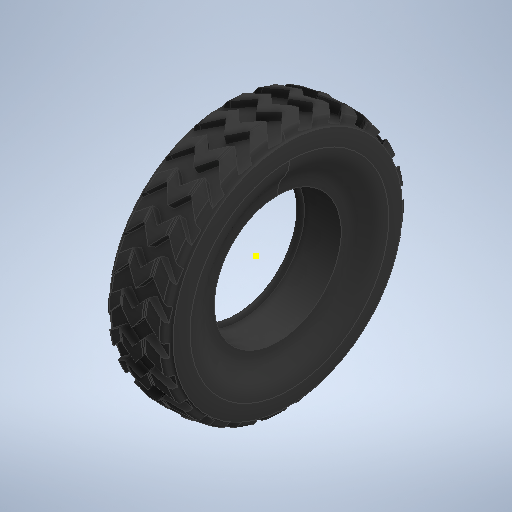
# Autodesk Inventor part: eg 243 tyre
Saved by Autodesk Inventor 2025 (Build 290162000, 162)
## iProperties
Created: 2024-11-03
Part Number: eg 243 tyre
Material: Generic
Document SubType Name: Modeling
Designer: Student
Density: 1 g/cm^3
Appearance: Default
Author: Student
Autodesk Inventor part; units mm, degrees
ref_plane "YZ Plane" through (0, 0, 0) normal (1, 0, 0) x (0, 1, 0)
ref_plane "XZ Plane" through (0, 0, 0) normal (0, 1, 0) x (-1, 0, 0)
sketch "Sketch1" plane through (0, 0, 0) normal (0, 0, 1) x (1, 0, 0)
  line L0 (65, 190) -> (-45, 190)
  arc A0 (75, 397) -> (-75, 397) centre (0, 49.4375) ccw
  arc A1 (-75, 397) -> (-100, 297.5) centre (110.505, 297.5) ccw
  spline S0 degree 4 poles (-100, 297.5) (-100, 283.0211) (-97.3443, 254.0633) (-65, 233.4367) (-65, 204.4789) (-65, 190) knots 0 0 0 0 0 0.5 1 1 1 1 1
  arc A2 (100, 297.5) -> (75, 397) centre (-110.505, 297.5) ccw
  arc A3 (-65, 190) -> (-45, 190) centre (-55, 190) ccw
  line L1 (-45, 190) -> (65, 190)
  line L2 (-75, 0) -> (75, 0)
  line L3 (65, 190) -> (65, 219.4167)
  spline S1 degree 4 poles (100, 297.5) (100, 283.0211) (97.3443, 254.0633) (65, 233.4367) (65, 204.4789) (65, 190) knots 0 0 0 0 0 0.5 1 1 1 1 1
  point P0 (0, 0)
  dimension "d11" = 20
  constraints: 8 end point, 8 point on circle, 4 centre point, 2 vertical, 1 collinear, 1 horizontal, 7 other
  measures "d11" distance of A3.start L0.end
revolve "Revolution1" add sketch "Sketch1" angle 360 about axis through (-75, 0, 0) along (1, 0, 0)
sketch "Sketch2" plane through (0, 0, 0) normal (0, 0, 1) x (1, 0, 0)
  line L0 (0, 0) -> (0, 447.3239)
  line L1 (0, 0) -> (252.2456, 0)
  line L2 (-125.0211, 343.2156) -> (-94.976, 343.2156)
  arc A0 (-75, 397) -> (-100, 297.5) centre (110.505, 297.5) ccw projected
  line L3 (-75, -397) -> (-75, 397) projected
  line L4 (-75, 364.2118) -> (-38.26, 370.6901)
  arc A1 (-38.26, 370.6901) -> (-34.9982, 371.8769) centre (-39.9965, 380.5381) ccw
  arc A2 (-30, 373.2156) -> (-34.9982, 371.8769) centre (-30, 363.2156) ccw
  line L5 (-30, 373.2156) -> (0, 373.2156)
  spline S0 degree 4 poles (-94.976, 343.2156) (-90.7906, 343.2156) (-82.4198, 343.2156) (-86.7482, 362.1403) (-78.9161, 363.5213) (-75, 364.2118) knots 0 0 0 0 0 0.5 1 1 1 1 1
  line L6 (125.0211, 343.2156) -> (94.976, 343.2156)
  line L7 (75, 364.2118) -> (38.26, 370.6901)
  arc A3 (34.9982, 371.8769) -> (38.26, 370.6901) centre (39.9965, 380.5381) ccw
  arc A4 (34.9982, 371.8769) -> (30, 373.2156) centre (30, 363.2156) ccw
  line L8 (30, 373.2156) -> (0, 373.2156)
  spline S1 degree 4 poles (94.976, 343.2156) (90.7906, 343.2156) (82.4198, 343.2156) (86.7482, 362.1403) (78.9161, 363.5213) (75, 364.2118) knots 0 0 0 0 0 0.5 1 1 1 1 1
  arc A5 (-75, 397) -> (-94.976, 343.2156) centre (110.505, 297.5) ccw
  arc A6 (75, 397) -> (-75, 397) centre (0, 49.4375) ccw projected
  arc A7 (75, 397) -> (-75, 397) centre (0, 49.4375) ccw
  arc A8 (94.976, 343.2156) -> (75, 397) centre (-110.505, 297.5) ccw
  dimension "d14" = 30
  dimension "d15" = 10
  dimension "d17" = 10
  dimension "d18" = 76.52
  dimension "d19" = 170
  dimension "d20" = 30
  constraints: 16 end point, 16 point on circle, 8 symmetric about line, 7 centre point, 4 horizontal, 3 tangent, 2 point on line, 1 concentric, 1 perpendicular, 1 vertical, 8 other
  measures "d14" distance of L5.start L5.end
  measures "d15" radius of A2
  measures "d17" radius of A1
  measures "d18" diameter of L4.end L0
  measures "d19" angle of L5 L4
  measures "d20" distance between parallel lines of L5 L2
sketch "Sketch3" plane through (0, 0, 0) normal (0, 0, 1) x (1, 0, 0)
  point P0 (0, 0)
revolve "Revolution2" cut sketch "Sketch2" angle 360 about axis through (0, 0, 0) along (1, 0, 0)
ref_plane "Work Plane1" through (0, 0, 375) normal (0, 0, 1) x (1, 0, 0)
sketch "Sketch4" plane through (0, 0, 375) normal (0, 0, 1) x (1, 0, 0)
  line L0 (-75, 364.2118) -> (-75, -364.2118) projected
  line L1 (-75, 0) -> (-34.9982, 44.3766)
  line L2 (-34.9982, 371.8769) -> (-34.9982, -371.8769) projected
  line L3 (0, 0) -> (-34.9982, 44.3766)
  line L4 (0, 0) -> (34.9982, 44.3766)
  line L5 (34.9982, 371.8769) -> (34.9982, -371.8769) projected
  line L6 (34.9982, 44.3766) -> (75, 0)
  line L7 (75, 364.2118) -> (75, -364.2118) projected
  line L8 (75, -39.6254) -> (38.26, -6.5074)
  line L9 (38.26, 370.6901) -> (38.26, -370.6901) projected
  line L10 (38.26, -6.5074) -> (0, -48.9518)
  line L11 (0, -48.9518) -> (-34.9982, -17.4038)
  line L12 (-75, -48.9518) -> (-34.9982, -17.4038)
  line L13 (-75, 0) -> (-100, -27.7296)
  line L14 (-100, -297.5) -> (-100, 297.5) projected
  line L15 (-75, -48.9518) -> (-100, -68.6684)
  line L16 (-100, -68.6684) -> (-100, -27.7296)
  line L17 (75, 0) -> (110.5161, -33.1778)
  line L18 (110.5161, -33.1778) -> (110.5161, -68.6684)
  line L19 (75, -39.6254) -> (110.5161, -71.6402)
  line L20 (110.5161, -71.6402) -> (110.5161, -33.1778)
  line L21 (-100, -27.7296) -> (-100, -68.6684)
  constraints: 32 end point, 8 point on line, 3 collinear, 2 midpoint, 1 perpendicular, 1 vertical
extrude "Extrusion1" cut sketch "Sketch4" against normal blind 30
pattern_circular "Circular Pattern1" count 24 over 360 about axis through (-10, 0, 0) along (1, 0, 0) of "Extrusion1"
body "Solid1"
